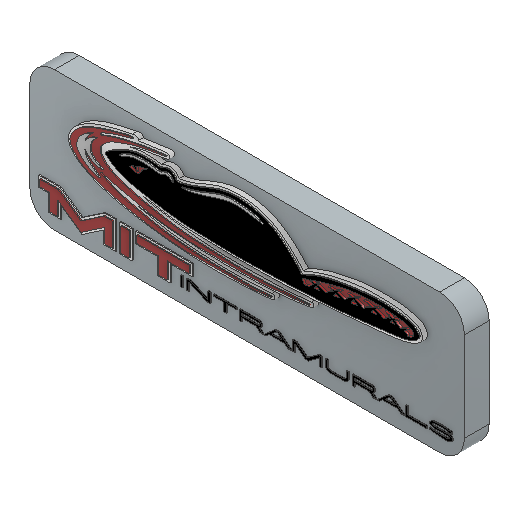
# Autodesk Inventor part: MIT Intramurals Banner
Saved by Autodesk Inventor 2026.2 (Build 302298000, 298)
## iProperties
Created: 2025-12-23
Part Number: MIT Intramurals Banner
Material: Generic
Document SubType Name: Modeling
Designer: andyeske
Density: 1 g/cm^3
Appearance: Default
Author: andyeske
Autodesk Inventor part; units mm, degrees
(part 1 of 2)
ref_plane "YZ Plane" through (0, 0, 0) normal (1, 0, 0) x (0, 1, 0)
ref_plane "XZ Plane" through (0, 0, 0) normal (0, 1, 0) x (-1, 0, 0)
ref_plane "XY Plane" through (0, 0, 0) normal (0, 0, 1) x (1, 0, 0)
sketch "Sketch1" plane through (0, 0, 0) normal (0, 0, 1) x (1, 0, 0)
  line L0 (-102.5583, 25.4534) -> (110.5342, 25.4534) construction
  line L1 (110.5342, 25.4534) -> (110.5342, -35.8107) construction
  line L2 (110.5342, -35.8107) -> (-102.5583, -35.8107) construction
  line L3 (-102.5583, -35.8107) -> (-102.5583, 25.4534) construction
  line L4 (-102.5583, 25.4534) -> (110.5342, 25.4534) construction
  line L5 (110.5342, 25.4534) -> (110.5342, -35.8107) construction
  line L6 (110.5342, -35.8107) -> (-102.5583, -35.8107) construction
  line L7 (-102.5583, -35.8107) -> (-102.5583, 25.4534) construction
  line L8 (-102.5583, -5.1786) -> (110.5342, -5.1786) construction
  line L9 (-107.6383, -40.8907) -> (115.6142, -40.8907)
  line L10 (115.6142, -40.8907) -> (115.6142, 30.5334)
  line L11 (115.6142, 30.5334) -> (-107.6383, 30.5334)
  line L12 (-107.6383, 30.5334) -> (-107.6383, -40.8907)
  line L13 (-107.6383, -40.8907) -> (115.6142, 30.5334) construction
  line L14 (115.6142, -40.8907) -> (-107.6383, 30.5334) construction
  spline S0 degree 4 poles (-52.4492, 24.3714) (-58.8702, 22.9595) (-67.573, 21.6476) (-80.0555, 16.5547) (-86.0471, 8.2755) (-85.3196, 1.057) (-71.5894, -7.0587) (-54.9195, -10.8267) (-25.8271, -15.277) (-1.6342, -15.5021) (17.3081, -13.4799) (19.6488, -13.3581) knots 0 0 0 0 0 0.204161 0.274872 0.345733 0.425063 0.520803 0.635182 0.756576 1 1 1 1 1
  spline S1 degree 4 poles (-49.0567, -6.4057) (-39.7782, -7.8854) (-36.8573, -10.6647) (4.3156, -12.1007) (6.0375, -11.212) (19.2729, -10.6088) knots 0 0 0 0 0 0.481309 1 1 1 1 1
  spline S2 degree 4 poles (-48.9231, -6.0144) (-47.2856, -6.3603) (-30.209, -9.1125) (-6.7858, -10.1005) (21.0365, -9.6313) (34.1993, -7.9209) (39.788, -6.6471) knots 0 0 0 0 0 0.386042 0.578559 1 1 1 1 1
  spline S3 degree 4 poles (-46.5779, -0.655) (-43.8171, -2.1998) (-20.6221, -4.7597) (-12.4054, -6.1125) (7.8539, -5.9766) (21.1432, -5.4197) (30.3375, -5.6283) (37.164, -4.3462) (39.6442, -4.2865) knots 0 0 0 0 0 0.358399 0.500414 0.629553 0.752083 1 1 1 1 1
  spline S4 degree 4 poles (-46.5779, -0.428) (-40.6413, -0.834) (-35.092, -3.6944) (-11.838, -3.5836) (9.8953, -4.1536) (37.76, -3.0641) (49.5551, -1.9589) (82.2104, 0.7181) (92.0004, 2.7859) (96.3774, 6.0719) (96.9345, 8.5326) (95.573, 12.2204) (91.8952, 13.5262) (86.96, 14.8593) (82.3457, 15.5732) (74.0371, 15.7321) (67.2255, 15.6466) (59.1842, 14.6025) (48.4661, 12.069) (45.437, 11.6483) (35.3646, 7.4843) (35.471, 7.4588) knots 0 0 0 0 0 0.13521 0.204072 0.278186 0.357458 0.429675 0.488839 0.535364 0.566154 0.593435 0.622619 0.655256 0.692209 0.732593 0.775833 0.821274 0.864817 0.909076 1 1 1 1 1
  spline S5 degree 4 poles (35.471, 7.4588) (32.9093, 10.589) (24.1083, 20.0316) (15.0532, 23.4669) (4.122, 25.3465) (-4.4474, 24.7856) (-11.5501, 22.5181) (-21.6412, 18.1562) (-21.1605, 18.2177) (-27.5995, 16.4904) (-28.3232, 16.6931) knots 0 0 0 0 0 0.300543 0.415952 0.52752 0.636808 0.734219 0.82255 1 1 1 1 1
  spline S6 degree 4 poles (-28.3232, 16.6931) (-29.0007, 17.4703) (-29.5286, 18.6185) (-32.267, 20.3015) (-35.437, 19.4052) (-36.852, 18.6173) (-37.322, 18.4594) knots 0 0 0 0 0 0.41933 0.600199 1 1 1 1 1
  spline S7 degree 4 poles (-37.322, 18.4594) (-38.5691, 18.5544) (-43.1872, 19.8396) (-49.0015, 18.9635) (-52.3655, 18.5024) (-53.4631, 18.0644) knots 0 0 0 0 0 0.521417 1 1 1 1 1
  spline S8 degree 4 poles (-53.5099, 18.2245) (-50.9519, 19.1283) (-47.5068, 20.3499) (-40.9121, 20.7668) (-34.7831, 22.3278) (-33.7292, 22.3321) (-33.0986, 23.0952) (-32.9733, 24.2409) (-33.4725, 24.8827) (-35.3883, 25.1437) (-39.835, 24.1062) (-46.9335, 23.5297) (-47.4631, 23.1662) (-49.3709, 23.0321) knots 0 0 0 0 0 0.266365 0.357545 0.430443 0.483452 0.524772 0.568835 0.624773 0.699993 0.786792 1 1 1 1 1
  spline S9 degree 4 poles (-49.3709, 23.0321) (-49.3469, 23.256) (-49.3072, 24.335) (-49.9777, 24.9683) (-51.9566, 24.5536) (-52.4492, 24.3714) knots 0 0 0 0 0 0.425634 1 1 1 1 1
  arc A0 (19.6488, -13.3581) -> (19.2729, -10.6088) centre (19.4518, -11.9847) ccw
  arc A1 (39.788, -6.6471) -> (39.6442, -4.2865) centre (39.6727, -5.4694) ccw
  arc A2 (-48.9231, -6.0144) -> (-49.0567, -6.4057) centre (-48.9661, -6.2182) ccw
  arc A3 (-46.5779, -0.428) -> (-46.5779, -0.655) centre (-46.5512, -0.5415) ccw
  arc A4 (-53.5099, 18.2245) -> (-53.4631, 18.0644) centre (-53.4821, 18.1458) ccw
  spline S10 degree 4 poles (-71.97, 15.4745) (-73.5618, 14.8176) (-78.0389, 12.5988) (-80.1652, 8.5391) (-80.3177, 3.0778) (-71.7488, -2.2177) (-71.8816, -1.1731) (-68.0997, -2.6081) knots 0 0 0 0 0 0.349269 0.493319 0.634154 1 1 1 1 1
  spline S11 degree 3 poles (-71.97, 15.4745) (-73.2885, 14.039) (-75.2326, 12.8836) (-75.6158, 10.3382) knots 0 0 0 0 1 1 1 1
  spline S12 degree 3 poles (-75.6158, 10.3382) (-74.6308, 12.2137) (-72.1942, 13.8735) (-69.6154, 14.6163) knots 0 0 0 0 1 1 1 1
  spline S13 degree 4 poles (-69.6154, 14.6163) (-70.4759, 13.8231) (-72.3788, 12.3221) (-73.059, 10.2756) (-73.1664, 5.2191) (-69.7067, 3.7408) (-68.2199, 2.6138) (-66.4762, 1.8118) knots 0 0 0 0 0 0.339065 0.480526 0.625412 1 1 1 1 1
  spline S14 degree 4 poles (-75.8015, 6.7353) (-74.6191, 4.6802) (-72.4475, 2.5037) (-68.6605, 1.822) (-66.4762, 1.8118) knots 0 0 0 0 0 1 1 1 1 1
  spline S15 degree 4 poles (-75.8015, 6.7353) (-75.5788, 4.044) (-75.7088, 2.5492) (-69.058, -1.4354) (-68.0997, -2.6081) knots 0 0 0 0 0 1 1 1 1 1
  spline S16 degree 4 poles (-52.048, 23.4288) (-54.2401, 23.3528) (-66.6857, 19.9381) (-79.4427, 16.3789) (-84.3823, 7.744) (-84.209, 4.7623) (-78.8244, -2.3227) (-66.6046, -6.5374) (-51.6417, -10.096) (-41.0552, -11.7905) (-18.7063, -14.7429) (-1.7175, -12.2275) (3.8289, -14.3334) (19.2729, -12.2118) knots 0 0 0 0 0 0.18081 0.244398 0.299004 0.356886 0.425964 0.50631 0.595714 0.686149 0.771857 1 1 1 1 1
  spline S17 degree 4 poles (-51.972, 22.8466) (-57.6402, 21.3754) (-58.1641, 21.4536) (-67.5415, 18.1413) (-68.4686, 17.0097) knots 0 0 0 0 0 1 1 1 1 1
  spline S18 degree 4 poles (-67.7151, 16.4274) (-64.426, 17.854) (-60.1317, 19.3505) (-45.9619, 22.8498) (-40.2437, 23.0375) (-34.715, 23.8652) knots 0 0 0 0 0 0.467692 1 1 1 1 1
  spline S19 degree 4 poles (-34.6772, 23.4704) (-38.4839, 22.7648) (-40.4639, 22.3554) (-50.7282, 21.246) (-60.3841, 16.8007) (-62.8171, 16.4662) (-68.298, 12.2075) (-69.5248, 8.3693) (-64.0493, 2.7683) (-55.3104, -0.0117) (-47.7069, -2.169) (-33.9304, -4.8768) (-23.6731, -6.2287) (-9.6141, -6.7589) (3.746, -7.4013) (15.6562, -7.092) (30.638, -6.3684) (37.5145, -5.6068) (39.0554, -5.469) knots 0 0 0 0 0 0.119852 0.168842 0.217962 0.26068 0.302266 0.349885 0.400894 0.460541 0.525181 0.593374 0.664659 0.734215 0.804927 0.871867 1 1 1 1 1
  spline S20 degree 4 poles (39.108, -5.7709) (37.4385, -6.308) (23.1011, -7.5786) (13.1163, -8.7313) (-7.0091, -8.2583) (-21.4952, -8.578) (-29.5439, -7.3415) (-41.2987, -6.7959) (-48.8299, -4.501) (-65.2605, -1.3176) (-67.5791, 0.1162) knots 0 0 0 0 0 0.240077 0.356564 0.466749 0.569739 0.662256 0.754281 1 1 1 1 1
  spline S21 degree 4 poles (-68.0997, -0.655) (-62.5259, -3.4157) (-61.765, -4.6975) (-42.4071, -9.0657) (-34.3124, -10.69) (-17.9846, -11.881) (-11.8888, -12.3355) (4.7444, -12.3507) (10.0463, -12.6177) (17.9731, -11.9242) (19.2729, -11.797) knots 0 0 0 0 0 0.246404 0.35873 0.472789 0.584911 0.695079 0.795942 1 1 1 1 1
  arc A5 (19.2729, -12.2118) -> (19.2729, -11.797) centre (19.2444, -12.0044) ccw
  arc A6 (-67.5791, 0.1162) -> (-68.0997, -0.655) centre (-67.7515, -0.3288) ccw
  arc A7 (39.108, -5.7709) -> (39.0554, -5.469) centre (39.0691, -5.6221) ccw
  arc A8 (-51.972, 22.8466) -> (-52.048, 23.4288) centre (-52.0378, 23.1341) ccw
  arc A9 (-34.6772, 23.4704) -> (-34.715, 23.8652) centre (-34.6856, 23.6688) ccw
  spline S22 degree 4 poles (-65.879, 9.2635) (-65.8749, 11.3275) (-55.3373, 15.7109) (-53.6712, 18.2111) (-38.9955, 17.9177) (-37.405, 16.714) (-33.7493, 19.5352) (-31.3534, 18.3976) (-29.5789, 16.7809) (-29.4647, 15.575) knots 0 0 0 0 0 0.357646 0.495506 0.61467 0.716133 0.79801 1 1 1 1 1
  spline S23 degree 4 poles (-29.4647, 15.575) (-28.1519, 15.0835) (-24.5872, 15.8727) (-18.5009, 18.1038) (-12.5083, 20.6718) (-6.1161, 23.2421) (3.0018, 24.3814) (11.5231, 23.0257) (21.4229, 19.5107) (27.5772, 14.3886) (34.927, 6.7369) (34.8654, 5.7735) knots 0 0 0 0 0 0.174571 0.259653 0.353316 0.452487 0.556196 0.662312 0.769869 1 1 1 1 1
  spline S24 degree 4 poles (34.8654, 5.7735) (40.8292, 8.1161) (40.6549, 10.0927) (71.7532, 15.7804) (83.2327, 13.7336) (92.5145, 13.0285) (96.6582, 8.6519) (94.223, 5.852) (89.2683, 3.6409) (84.9003, 2.9408) (72.4496, 1.6108) (62.4885, 0.1154) (50.6338, -0.6616) (26.6259, -2.1909) (16.6731, -2.1299) (2.2887, -2.9635) (-18.4876, -2.0158) (-30.9684, -1.9125) (-54.5772, 2.6604) (-59.4474, 3.6818) (-65.879, 9.2635) knots 0 0 0 0 0 0.126651 0.181647 0.230811 0.266967 0.298491 0.327835 0.362864 0.404742 0.452577 0.510294 0.568494 0.62822 0.690828 0.748447 0.808493 0.867431 1 1 1 1 1
  spline S25 degree 4 poles (-58.3596, 12.6825) (-57.2325, 13.7843) (-51.9107, 17.5748) (-41.5573, 16.8573) (-38.56, 15.7519) (-36.7348, 15.5391) (-35.2387, 16.9945) (-32.33, 17.386) (-31.3664, 15.6515) (-30.3695, 15.3825) (-30.6352, 13.9476) knots 0 0 0 0 0 0.357484 0.480034 0.576415 0.657357 0.736723 0.814996 1 1 1 1 1
  spline S26 degree 4 poles (-30.6352, 13.9476) (-30.9382, 14.2243) (-32.1883, 16.178) (-34.3185, 16.1348) (-36.0839, 15.0225) (-37.1207, 14.3376) (-39.694, 14.8986) (-41.6476, 15.3507) (-45.7698, 15.473) (-50.3637, 15.66) (-54.9604, 14.1617) (-57.2368, 12.3666) (-58.3596, 12.6825) knots 0 0 0 0 0 0.170055 0.237891 0.305971 0.377561 0.459955 0.555332 0.659577 0.768342 1 1 1 1 1
  spline S27 degree 4 poles (-26.2639, 14.356) (-23.3906, 14.8149) (-14.9027, 16.789) (-5.1775, 24.2035) (8.399, 20.9689) (12.1626, 21.0227) (15.3623, 18.6573) knots 0 0 0 0 0 0.432201 0.610065 1 1 1 1 1
  spline S28 degree 4 poles (15.3623, 18.6573) (14.0844, 19.1095) (6.0457, 20.2504) (1.0033, 21.6252) (-13.688, 16.6903) (-14.6354, 16.5131) (-24.8081, 13.4817) (-26.2639, 14.356) knots 0 0 0 0 0 0.34942 0.500031 0.649154 1 1 1 1 1
  spline S29 degree 2 poles (-53.3008, 9.911) (-52.5867, 10.6807) (-51.5889, 11.0921) knots 0 0 0 1 1 1
  line L15 (-51.5889, 11.0921) -> (-49.9017, 9.2326)
  line L16 (-49.9017, 9.2326) -> (-50.0556, 11.6422)
  spline S30 degree 3 poles (-50.0556, 11.6422) (-48.6963, 12.1055) (-46.1374, 12.8984) (-44.3311, 13.1726) knots 0 0 0 0 1 1 1 1
  spline S31 degree 3 poles (-44.3311, 13.1726) (-45.5318, 12.4854) (-46.2357, 11.5206) (-47.2677, 11.1827) knots 0 0 0 0 1 1 1 1
  spline S32 degree 4 poles (-47.2677, 11.1827) (-47.3636, 10.8042) (-47.2649, 10.0321) (-49.615, 8.1093) (-50.6841, 8.6477) (-52.7122, 9.4891) (-53.3008, 9.911) knots 0 0 0 0 0 0.361372 0.533494 1 1 1 1 1
  line L17 (35.2952, 4.3814) -> (36.3498, 1.9636)
  spline S33 degree 2 poles (35.2952, 4.3814) (37.0043, 5.036) (38.6042, 5.5033) knots 0 0 0 1 1 1
  spline S34 degree 2 poles (36.3498, 1.9636) (37.741, 2.2189) (38.9714, 2.5521) knots 0 0 0 1 1 1
  spline S35 degree 2 poles (38.9714, 2.5521) (39.7159, 3.5541) (41.2291, 4.6206) knots 0 0 0 1 1 1
  spline S36 degree 2 poles (38.6042, 5.5033) (40.0266, 5.3532) (41.2291, 4.6206) knots 0 0 0 1 1 1
  spline S37 degree 2 poles (39.2749, 5.685) (40.8676, 5.5413) (42.1574, 5.2848) knots 0 0 0 1 1 1
  spline S38 degree 4 poles (39.2749, 5.685) (40.1857, 6.0134) (43.263, 7.1325) (47.2971, 8.314) (55.8577, 10.4813) (59.3016, 11.343) (70.558, 12.3008) (76.0447, 12.4509) (85.7728, 11.2662) (89.5634, 10.9909) (92.783, 8.8272) (92.8791, 7.6694) (92.0215, 6.1081) (89.9165, 5.6648) (89.4278, 5.5033) knots 0 0 0 0 0 0.162413 0.243574 0.336675 0.435958 0.540053 0.643161 0.731074 0.799741 0.849228 0.891651 1 1 1 1 1
  spline S39 degree 3 poles (89.4278, 5.5033) (90.0048, 6.3278) (88.6176, 6.9599) (87.5827, 7.1374) knots 0 0 0 0 1 1 1 1
  spline S40 degree 2 poles (87.5827, 7.1374) (88.251, 8.0136) (89.9993, 8.7444) knots 0 0 0 1 1 1
  spline S41 degree 3 poles (89.9993, 8.7444) (89.0353, 9.1151) (87.0785, 8.2126) (85.9445, 7.2852) knots 0 0 0 0 1 1 1 1
  spline S42 degree 2 poles (85.9445, 7.2852) (85.1544, 8.1452) (82.7618, 9.2635) knots 0 0 0 1 1 1
  spline S43 degree 2 poles (82.7618, 9.2635) (83.5886, 10.0911) (85.0626, 10.3382) knots 0 0 0 1 1 1
  spline S44 degree 2 poles (85.0626, 10.3382) (83.7496, 10.5873) (81.9313, 9.718) knots 0 0 0 1 1 1
  spline S45 degree 3 poles (81.9313, 9.718) (80.9342, 10.2789) (79.3639, 10.9061) (77.8217, 11.0035) knots 0 0 0 0 1 1 1 1
  spline S46 degree 3 poles (77.8217, 11.0035) (78.7555, 10.5207) (80.1921, 9.8801) (80.6667, 9.2635) knots 0 0 0 0 1 1 1 1
  spline S47 degree 3 poles (80.6667, 9.2635) (78.9368, 8.8382) (78.6712, 8.3465) (77.423, 7.4588) knots 0 0 0 0 1 1 1 1
  spline S48 degree 2 poles (80.6667, 7.5944) (80.9598, 8.3322) (81.6868, 8.7444) knots 0 0 0 1 1 1
  spline S49 degree 2 poles (81.6868, 8.7444) (82.2926, 8.3928) (82.8551, 7.5944) knots 0 0 0 1 1 1
  line L18 (80.6667, 7.5944) -> (82.8551, 7.5944)
  line L19 (70.7025, 7.1374) -> (73.8247, 7.2162)
  line L20 (60.3527, 5.9944) -> (63.8972, 6.3408)
  line L21 (51.5538, 4.7315) -> (54.4025, 5.2848)
  line L22 (41.6408, 3.0069) -> (44.1266, 3.4055)
  spline S50 degree 2 poles (41.6408, 3.0069) (41.951, 3.9202) (42.3855, 4.2937) knots 0 0 0 1 1 1
  spline S51 degree 2 poles (42.3855, 4.2937) (43.4958, 4.1245) (44.1266, 3.4055) knots 0 0 0 1 1 1
  spline S52 degree 2 poles (42.1574, 5.2848) (43.1477, 6.2989) (44.8399, 7.0186) knots 0 0 0 1 1 1
  spline S53 degree 2 poles (44.8399, 7.0186) (43.7611, 6.1187) (43.1407, 5.2848) knots 0 0 0 1 1 1
  spline S54 degree 3 poles (43.1407, 5.2848) (44.4101, 5.0932) (46.3814, 4.5665) (47.5565, 4.0873) knots 0 0 0 0 1 1 1 1
  spline S55 degree 3 poles (47.5565, 4.0873) (48.3925, 4.8563) (50.3732, 6.2541) (51.2037, 6.5341) knots 0 0 0 0 1 1 1 1
  spline S56 degree 3 poles (51.2037, 6.5341) (50.1722, 6.995) (49.7103, 7.113) (48.5739, 7.2608) knots 0 0 0 0 1 1 1 1
  spline S57 degree 3 poles (48.5739, 7.2608) (49.332, 7.5631) (51.2725, 7.4257) (52.024, 7.099) knots 0 0 0 0 1 1 1 1
  spline S58 degree 3 poles (52.024, 7.099) (53.0571, 7.7103) (54.2865, 8.498) (55.7131, 8.7927) knots 0 0 0 0 1 1 1 1
  spline S59 degree 3 poles (55.7131, 8.7927) (54.9237, 8.3987) (53.6734, 7.6255) (53.2188, 7.0186) knots 0 0 0 0 1 1 1 1
  spline S60 degree 3 poles (53.2188, 7.0186) (53.9015, 6.9339) (55.7193, 6.6122) (56.9696, 5.685) knots 0 0 0 0 1 1 1 1
  spline S61 degree 2 poles (51.5538, 4.7315) (51.7348, 5.3219) (52.4733, 6.2312) knots 0 0 0 1 1 1
  spline S62 degree 2 poles (52.4733, 6.2312) (53.4059, 5.9476) (54.4025, 5.2848) knots 0 0 0 1 1 1
  spline S63 degree 2 poles (70.7025, 7.1374) (71.1539, 7.9459) (72.0142, 8.5077) knots 0 0 0 1 1 1
  spline S64 degree 2 poles (72.0142, 8.5077) (73.1907, 8.178) (73.8247, 7.2162) knots 0 0 0 1 1 1
  spline S65 degree 2 poles (60.3527, 5.9944) (60.8212, 7.1738) (61.7016, 8.0103) knots 0 0 0 1 1 1
  spline S66 degree 2 poles (61.7016, 8.0103) (63.1746, 7.5515) (63.8972, 6.3408) knots 0 0 0 1 1 1
  spline S67 degree 2 poles (56.9696, 5.685) (58.6077, 7.5518) (60.7559, 8.5077) knots 0 0 0 1 1 1
  spline S68 degree 2 poles (60.7559, 8.5077) (59.8431, 8.9671) (58.568, 9.2635) knots 0 0 0 1 1 1
  spline S69 degree 2 poles (58.568, 9.2635) (59.9688, 9.4306) (61.5188, 8.9027) knots 0 0 0 1 1 1
  spline S70 degree 2 poles (61.5188, 8.9027) (62.6832, 9.7229) (64.527, 10.2202) knots 0 0 0 1 1 1
  spline S71 degree 2 poles (64.527, 10.2202) (63.4518, 9.6666) (62.5551, 8.7927) knots 0 0 0 1 1 1
  spline S72 degree 3 poles (62.5551, 8.7927) (64.4258, 8.2771) (65.688, 7.6378) (66.7581, 6.7295) knots 0 0 0 0 1 1 1 1
  spline S73 degree 3 poles (66.7581, 6.7295) (67.8827, 7.847) (69.6665, 8.8024) (70.7025, 8.9027) knots 0 0 0 0 1 1 1 1
  spline S74 degree 3 poles (70.7025, 8.9027) (70.1912, 9.604) (68.038, 10.1459) (66.9267, 10.338) knots 0 0 0 0 1 1 1 1
  spline S75 degree 3 poles (66.9267, 10.338) (68.3767, 10.6734) (70.5215, 9.7878) (71.7293, 9.5928) knots 0 0 0 0 1 1 1 1
  spline S76 degree 3 poles (71.7293, 9.5928) (72.6223, 9.9336) (74.2672, 10.8902) (75.4899, 10.9318) knots 0 0 0 0 1 1 1 1
  spline S77 degree 3 poles (75.4899, 10.9318) (74.5963, 10.619) (73.0858, 9.6113) (72.8404, 9.2635) knots 0 0 0 0 1 1 1 1
  spline S78 degree 3 poles (72.8404, 9.2635) (74.6153, 8.8325) (75.731, 8.1456) (77.423, 7.4588) knots 0 0 0 0 1 1 1 1
  line L23 (-101.4437, -24.341) -> (-96.395, -24.341)
  line L24 (-96.395, -24.341) -> (-96.395, -32.9519)
  line L25 (-96.395, -32.9519) -> (-92.1637, -32.9519)
  line L26 (-92.1637, -32.9519) -> (-92.1637, -25.7224)
  line L27 (-92.1637, -25.7224) -> (-80.2835, -34.0057)
  line L28 (-80.2835, -34.0057) -> (-68.147, -25.7224)
  line L29 (-68.147, -25.7224) -> (-68.147, -33.1318)
  line L30 (-68.147, -33.1318) -> (-63.961, -33.1318)
  line L31 (-63.961, -33.1318) -> (-63.961, -20.8988)
  line L32 (-63.961, -20.8988) -> (-68.4676, -20.8988)
  line L33 (-68.4676, -20.8988) -> (-80.2835, -28.9632)
  line L34 (-80.2835, -28.9632) -> (-91.8499, -20.8988)
  line L35 (-91.8499, -20.8988) -> (-101.4437, -20.8988)
  line L36 (-101.4437, -20.8988) -> (-101.4437, -24.341)
  line L37 (-59.868, -20.8988) -> (-55.6283, -20.8988)
  line L38 (-55.6283, -20.8988) -> (-55.6283, -33.1318)
  line L39 (-55.6283, -33.1318) -> (-59.868, -33.1318)
  line L40 (-59.868, -33.1318) -> (-59.868, -20.8988)
  line L41 (-29.8009, -28.0712) -> (-28.5736, -28.0712)
  line L42 (-28.5736, -28.0712) -> (-28.5736, -33.1318)
  line L43 (-28.5736, -33.1318) -> (-29.8009, -33.1318)
  line L44 (-29.8009, -33.1318) -> (-29.8009, -28.0712)
  line L45 (-51.7454, -20.8988) -> (-51.7454, -24.6191)
  line L46 (-51.7454, -24.6191) -> (-40.4236, -24.6191)
  line L47 (-40.4236, -24.6191) -> (-40.4236, -33.1318)
  line L48 (-40.4236, -33.1318) -> (-36.0253, -33.1318)
  line L49 (-36.0253, -33.1318) -> (-36.0253, -24.6191)
  line L50 (-36.0253, -24.6191) -> (-24.5946, -24.6191)
  line L51 (-24.5946, -24.6191) -> (-24.5946, -20.8988)
  line L52 (-24.5946, -20.8988) -> (-51.7454, -20.8988)
  line L53 (-26.5667, -28.0712) -> (-26.5667, -33.1318)
  line L54 (-26.5667, -33.1318) -> (-25.4696, -33.1318)
  line L55 (-25.4696, -33.1318) -> (-25.4696, -28.9632)
  line L56 (-25.4696, -28.9632) -> (-16.0059, -33.1318)
  line L57 (-16.0059, -33.1318) -> (-14.4445, -33.1318)
  line L58 (-14.4445, -33.1318) -> (-14.4445, -28.0712)
  line L59 (-14.4445, -28.0712) -> (-15.7205, -28.0712)
  line L60 (-15.7205, -28.0712) -> (-15.7205, -31.9239)
  line L61 (-15.7205, -31.9239) -> (-24.4669, -28.0712)
  line L62 (-24.4669, -28.0712) -> (-26.5667, -28.0712)
  line L63 (-12.884, -28.0712) -> (-0.8389, -28.0712)
  line L64 (-0.8389, -28.0712) -> (-0.8389, -28.9632)
  line L65 (-0.8389, -28.9632) -> (-6.1614, -28.9632)
  line L66 (-6.1614, -28.9632) -> (-6.1614, -33.1318)
  line L67 (-6.1614, -33.1318) -> (-7.5308, -33.1318)
  line L68 (-7.5308, -33.1318) -> (-7.5308, -28.9632)
  line L69 (-7.5308, -28.9632) -> (-12.884, -28.9632)
  line L70 (-12.884, -28.9632) -> (-12.884, -28.0712)
  line L71 (0.5155, -28.0712) -> (0.5155, -33.1318)
  line L72 (0.5155, -33.1318) -> (1.6717, -33.1318)
  line L73 (1.6717, -33.1318) -> (1.6717, -31.3271)
  line L74 (1.6717, -31.3271) -> (9.09, -31.3271)
  line L75 (9.09, -31.3271) -> (11.1121, -33.1318)
  line L76 (11.1121, -33.1318) -> (12.6994, -33.1318)
  line L77 (12.6994, -33.1318) -> (10.6774, -31.3271)
  line L78 (0.5155, -28.0712) -> (10.6774, -28.0712)
  line L79 (10.4286, -29.1342) -> (1.6717, -29.1342)
  line L80 (1.6717, -29.1342) -> (1.6717, -30.3018)
  line L81 (1.6717, -30.3018) -> (10.4286, -30.3018)
  arc A10 (10.4286, -30.3018) -> (10.4286, -29.1342) centre (10.3913, -29.718) ccw
  arc A11 (10.6774, -31.3271) -> (10.6774, -28.0712) centre (10.2386, -29.6991) ccw
  line L82 (12.9309, -33.1318) -> (18.7874, -28.0712)
  line L83 (18.7874, -28.0712) -> (20.8265, -28.0712)
  line L84 (20.8265, -28.0712) -> (27.1651, -33.1318)
  line L85 (27.1651, -33.1318) -> (25.5653, -33.1318)
  line L86 (25.5653, -33.1318) -> (23.734, -31.6698)
  line L87 (23.734, -31.6698) -> (15.8591, -31.6698)
  line L88 (15.8591, -31.6698) -> (14.1671, -33.1318)
  line L89 (14.1671, -33.1318) -> (12.9309, -33.1318)
  line L90 (17.1877, -30.7607) -> (22.4353, -30.7607)
  line L91 (22.4353, -30.7607) -> (20.4209, -28.798)
  line L92 (20.4209, -28.798) -> (19.4154, -28.798)
  line L93 (19.4154, -28.798) -> (17.1877, -30.7607)
  line L94 (172.9021, -50.0972) -> (-40.1904, -50.0972) construction
  line L95 (172.9021, -50.0972) -> (-40.1904, -50.0972) construction
  line L96 (58.6314, -28.0318) -> (58.6314, -33.0923)
  line L97 (58.6314, -33.0923) -> (59.7876, -33.0923)
  line L98 (59.7876, -33.0923) -> (59.7876, -31.2876)
  line L99 (59.7876, -31.2876) -> (67.2059, -31.2876)
  line L100 (67.2059, -31.2876) -> (69.228, -33.0923)
  line L101 (69.228, -33.0923) -> (70.8153, -33.0923)
  line L102 (70.8153, -33.0923) -> (68.7933, -31.2876)
  line L103 (58.6314, -28.0318) -> (68.7933, -28.0318)
  line L104 (68.5445, -29.0947) -> (59.7876, -29.0947)
  line L105 (59.7876, -29.0947) -> (59.7876, -30.2624)
  line L106 (59.7876, -30.2624) -> (68.5445, -30.2624)
  arc A12 (68.5445, -30.2624) -> (68.5445, -29.0947) centre (68.5073, -29.6785) ccw
  arc A13 (68.7933, -31.2876) -> (68.7933, -28.0318) centre (68.3545, -29.6597) ccw
  line L107 (71.0468, -33.0923) -> (76.9033, -28.0318)
  line L108 (76.9033, -28.0318) -> (78.9424, -28.0318)
  line L109 (78.9424, -28.0318) -> (85.281, -33.0923)
  line L110 (85.281, -33.0923) -> (83.6812, -33.0923)
  line L111 (83.6812, -33.0923) -> (81.8499, -31.6303)
  line L112 (81.8499, -31.6303) -> (73.975, -31.6303)
  line L113 (73.975, -31.6303) -> (72.2831, -33.0923)
  line L114 (72.2831, -33.0923) -> (71.0468, -33.0923)
  line L115 (75.3036, -30.7212) -> (80.5512, -30.7212)
  line L116 (80.5512, -30.7212) -> (78.5369, -28.7586)
  line L117 (78.5369, -28.7586) -> (77.5313, -28.7586)
  line L118 (77.5313, -28.7586) -> (75.3036, -30.7212)
  line L119 (27.6953, -33.0923) -> (27.6953, -28.0318)
  line L120 (27.6953, -28.0318) -> (29.6369, -28.0318)
  line L121 (29.6369, -28.0318) -> (35.2952, -32.19)
  line L122 (35.2952, -32.19) -> (41.2291, -28.0318)
  line L123 (41.2291, -28.0318) -> (42.8837, -28.0318)
  line L124 (42.8837, -28.0318) -> (42.8837, -33.0923)
  line L125 (42.8837, -33.0923) -> (41.6408, -33.0923)
  line L126 (41.6408, -33.0923) -> (41.6408, -29.0947)
  line L127 (41.6408, -29.0947) -> (36.1117, -33.3551)
  line L128 (36.1117, -33.3551) -> (34.439, -33.3551)
  line L129 (34.439, -33.3551) -> (29.0483, -29.1342)
  line L130 (29.0483, -29.1342) -> (29.0483, -33.0923)
  line L131 (29.0483, -33.0923) -> (27.6953, -33.0923)
  line L132 (44.5357, -28.0318) -> (45.8846, -28.0318)
  line L133 (44.5357, -28.0318) -> (44.5357, -31.2446)
  line L134 (45.8846, -28.0318) -> (45.8846, -31.2446)
  line L135 (55.4313, -31.1132) -> (55.4313, -28.0318)
  line L136 (55.4313, -28.0318) -> (56.7534, -28.0318)
  line L137 (56.7534, -28.0318) -> (56.7534, -31.1132)
  line L138 (47.9942, -32.19) -> (53.8931, -32.19)
  line L139 (47.4288, -33.0923) -> (54.2843, -33.0923)
  spline S79 degree 2 poles (45.8846, -31.2446) (46.106, -31.8542) (47.9942, -32.19) knots 0 0 0 1 1 1
  spline S80 degree 3 poles (44.5357, -31.2446) (44.5599, -32.2303) (45.931, -32.9686) (47.4288, -33.0923) knots 0 0 0 0 1 1 1 1
  spline S81 degree 3 poles (56.7534, -31.1132) (56.7847, -31.9085) (55.4171, -32.9141) (54.2843, -33.0923) knots 0 0 0 0 1 1 1 1
  spline S82 degree 2 poles (53.8931, -32.19) (55.2787, -31.9913) (55.4313, -31.1132) knots 0 0 0 1 1 1
  line L140 (85.9445, -28.0712) -> (87.1046, -28.0712)
  line L141 (87.1046, -28.0712) -> (87.1046, -31.9938)
  line L142 (87.1046, -31.9938) -> (96.8774, -31.9938)
  line L143 (96.8774, -31.9938) -> (96.8774, -33.0869)
  line L144 (96.8774, -33.0869) -> (85.9445, -33.0869)
  line L145 (85.9445, -33.0869) -> (85.9445, -28.0712)
  line L146 (98.2674, -31.6303) -> (98.2674, -32.5404)
  line L147 (109.6722, -28.4037) -> (109.6722, -29.3372)
  spline S83 degree 4 poles (109.6722, -28.4037) (108.7733, -28.0929) (105.6478, -27.7752) (103.1637, -27.669) (99.2636, -27.9958) (98.2311, -28.988) (98.1711, -29.9388) (99.4289, -31.0631) (101.7371, -30.9908) (105.1225, -30.9191) (107.0954, -30.7922) (108.598, -31.0126) (108.829, -31.6343) (107.9042, -32.2349) (105.4491, -32.1575) (101.0474, -32.2825) (98.7105, -31.9386) (98.2674, -31.6303) knots 0 0 0 0 0 0.176908 0.243948 0.300203 0.348723 0.396841 0.456186 0.523231 0.589094 0.644157 0.685091 0.722698 0.771731 0.835847 1 1 1 1 1
  spline S84 degree 4 poles (98.2674, -32.5404) (99.5553, -33.0936) (102.1491, -32.7939) (106.7339, -33.9297) (110.1842, -32.5353) (110.0663, -30.5611) (108.6148, -30.0593) (106.1535, -29.9773) (102.3534, -29.9259) (101.0004, -30.198) (99.2528, -29.843) (99.5332, -29.1911) (100.6421, -28.7892) (102.2414, -28.7031) (108.031, -28.4051) (107.7183, -29.2242) (109.6722, -29.3372) knots 0 0 0 0 0 0.193476 0.265024 0.326054 0.382919 0.447483 0.515446 0.581924 0.636535 0.67795 0.716326 0.766204 0.827883 1 1 1 1 1
  point P0 (0, 0)
  point P1 (3.9879, -5.1786)
  point P2 (-63.2696, 21.994)
  point P3 (-74.1898, 18.163)
  point P4 (-81.9273, 13.059)
  point P5 (-84.9907, 8.2462)
  point P6 (-84.46, 3.2243)
  point P7 (-75.3767, -4.2012)
  point P8 (-57.1798, -10.0522)
  point P9 (-32.848, -13.7119)
  point P10 (-6.16, -14.8406)
  point P11 (14.2841, -13.7934)
  point P12 (-39.1333, -8.3929)
  point P13 (-27.998, -10.0579)
  point P14 (-7.53, -11.2991)
  point P15 (5.0636, -11.3252)
  point P16 (-44.3448, -6.768)
  point P17 (-26.9622, -8.7993)
  point P18 (-6.5969, -9.7072)
  point P19 (14.2529, -9.4349)
  point P20 (30.7774, -8.1445)
  point P21 (-35.1237, -2.9829)
  point P22 (-16.8054, -5.1786)
  point P23 (-5.2292, -5.9063)
  point P24 (8.4022, -5.8766)
  point P25 (19.2472, -5.6046)
  point P26 (28.0274, -5.3492)
  point P27 (35.4082, -4.6884)
  point P28 (-39.5981, -1.5241)
  point P29 (-29.3179, -3.0262)
  point P30 (-10.4174, -3.7442)
  point P31 (10.1672, -3.8571)
  point P32 (34.8638, -3.027)
  point P33 (55.2915, -1.5051)
  point P34 (86.7801, 1.9619)
  point P35 (94.0802, 4.6158)
  point P36 (96.2193, 6.7261)
  point P37 (96.5848, 8.6266)
  point P38 (95.4548, 11.3806)
  point P39 (92.3217, 13.2998)
  point P40 (87.6339, 14.5956)
  point P41 (82.6419, 15.3745)
  point P42 (74.8311, 15.6746)
  point P43 (67.1736, 15.4606)
  point P44 (58.757, 14.3443)
  point P45 (51.1193, 12.7384)
  point P46 (45.883, 11.3954)
  point P47 (37.7337, 8.4225)
  point P48 (28.8398, 14.3559)
  point P49 (19.2717, 21.1238)
  point P50 (11.5307, 23.8652)
  point P51 (3.988, 24.9481)
  point P52 (-4.4388, 24.3714)
  point P53 (-13.1968, 21.7075)
  point P54 (-19.5689, 19.0248)
  point P55 (-21.7475, 18.1683)
  point P56 (-25.4696, 17.1317)
  point P57 (-29.2255, 17.8447)
  point P58 (-30.4143, 18.919)
  point P59 (-32.3677, 19.6364)
  point P60 (-34.677, 19.4695)
  point P61 (-36.5087, 18.8078)
  point P62 (-39.5897, 18.8083)
  point P63 (-44.0219, 19.2144)
  point P64 (-48.7169, 18.9607)
  point P65 (-51.8224, 18.5106)
  point P66 (-49.593, 19.473)
  point P67 (-44.0257, 20.5822)
  point P68 (-37.3281, 21.7165)
  point P69 (-34.2972, 22.3327)
  point P70 (-33.6058, 22.6038)
  point P71 (-33.1785, 23.201)
  point P72 (-33.0815, 24.0917)
  point P73 (-33.3977, 24.6171)
  point P74 (-34.5396, 24.9508)
  point P75 (-37.937, 24.6046)
  point P76 (-44.4064, 23.7068)
  point P77 (-47.4349, 23.2658)
  point P78 (-49.3615, 23.457)
  point P79 (-49.507, 24.0557)
  point P80 (-49.9521, 24.4922)
  point P81 (-51.1056, 24.6434)
  point P82 (-75.3651, 13.6542)
  point P83 (-78.6663, 10.4705)
  point P84 (-79.9317, 7.4588)
  point P85 (-79.5771, 4.6205)
  point P86 (-75.3649, 0.4414)
  point P87 (-71.9699, -1.3673)
  point P88 (-73.3328, 14.1502)
  point P89 (-74.7076, 12.6095)
  point P90 (-74.3626, 11.9588)
  point P91 (-72.2711, 13.4977)
  point P92 (-71.1635, 13.1726)
  point P93 (-72.4276, 11.4007)
  point P94 (-72.9824, 9.2635)
  point P95 (-72.7429, 6.6215)
  point P96 (-71.1254, 4.6206)
  point P97 (-68.9349, 3.1442)
  point P98 (-74.3628, 4.8608)
  point P99 (-71.9701, 3.1442)
  point P100 (-68.9349, 2.0854)
  point P101 (-75.5006, 4.7315)
  point P102 (-74.197, 2.5521)
  point P103 (-70.5188, -0.655)
  point P104 (-58.7239, 21.9977)
  point P105 (-73.5666, 17.1317)
  point P106 (-81.6263, 11.7004)
  point P107 (-83.8633, 7.7029)
  point P108 (-83.7541, 5.2058)
  point P109 (-80.2835, 0.4416)
  point P110 (-68.2715, -5.7102)
  point P111 (-52.4492, -9.7219)
  point P112 (-40.4236, -11.7967)
  point P113 (-24.7819, -13.3581)
  point P114 (-9.9687, -13.3581)
  point P115 (0.5155, -13.3581)
  point P116 (-56.7595, 21.6078)
  point P117 (-61.1409, 20.2417)
  point P118 (-66.4828, 18.1506)
  point P119 (-63.5422, 18.0643)
  point P120 (-58.2102, 19.6365)
  point P121 (-49.7373, 21.6078)
  point P122 (-42.2214, 22.8773)
  point P123 (-39.0088, 22.688)
  point P124 (-44.1604, 21.8246)
  point P125 (-53.849, 19.4702)
  point P126 (-60.4408, 17.0103)
  point P127 (-63.4115, 15.692)
  point P128 (-67.4906, 12.238)
  point P129 (-68.4656, 8.903)
  point P130 (-64.8238, 4.2941)
  point P131 (-56.5431, 0.442)
  point P132 (-47.8855, -1.9428)
  point P133 (-35.1146, -4.5144)
  point P134 (-23.4273, -6.0139)
  point P135 (-9.4628, -6.7901)
  point P136 (3.6455, -7.2272)
  point P137 (14.2708, -7.0717)
  point P138 (27.697, -6.4046)
  point P139 (36.5356, -5.7101)
  point P140 (34.1531, -6.5046)
  point P141 (21.1076, -7.7405)
  point P142 (8.4273, -8.3923)
  point P143 (-8.2602, -8.3913)
  point P144 (-22.5807, -8.1408)
  point P145 (-30.4198, -7.4265)
  point P146 (-37.3263, -6.7895)
  point P147 (-44.6879, -5.5691)
  point P148 (-58.2119, -2.6075)
  point P149 (-62.2204, -3.5962)
  point P150 (-54.9765, -6.0145)
  point P151 (-41.9684, -9.083)
  point P152 (-32.8492, -10.6082)
  point P153 (-19.1084, -11.7956)
  point P154 (-10.3187, -12.2468)
  point P155 (1.436, -12.3955)
  point P156 (9.341, -12.3982)
  point P157 (16.2097, -12.0534)
  point P158 (-62.3675, 12.4616)
  point P159 (-54.6455, 16.2882)
  point P160 (-47.3018, 17.8448)
  point P161 (-38.691, 17.4215)
  point P162 (-36.7676, 17.498)
  point P163 (-34.4878, 18.5117)
  point P164 (-32.3678, 18.5117)
  point P165 (-30.4181, 17.2972)
  point P166 (-27.3478, 15.4745)
  point P167 (-23.0284, 16.5574)
  point P168 (-17.6943, 18.5119)
  point P169 (-12.884, 20.4848)
  point P170 (-6.5796, 22.6878)
  point P171 (2.6728, 23.8652)
  point P172 (11.5307, 22.6878)
  point P173 (18.7874, 20.0395)
  point P174 (25.5653, 15.575)
  point P175 (33.007, 8.4244)
  point P176 (40.3926, 8.2429)
  point P177 (51.1245, 11.4007)
  point P178 (75.4899, 14.356)
  point P179 (86.3018, 13.4979)
  point P180 (93.6234, 11.1826)
  point P181 (95.4681, 8.4244)
  point P182 (94.2289, 6.3408)
  point P183 (90.4018, 4.2937)
  point P184 (85.6918, 3.1442)
  point P185 (74.8418, 1.8118)
  point P186 (63.7317, 0.4416)
  point P187 (50.5345, -0.655)
  point P188 (27.6953, -1.9432)
  point P189 (15.9178, -2.2996)
  point P190 (1.9042, -2.6081)
  point P191 (-17.3795, -2.1379)
  point P192 (-29.4647, -1.3672)
  point P193 (-45.8141, 1.1119)
  point P194 (-57.401, 3.9682)
  point P195 (-55.083, 14.786)
  point P196 (-45.73, 16.766)
  point P197 (-39.8397, 16.1558)
  point P198 (-38.1212, 15.7642)
  point P199 (-36.7882, 15.8656)
  dimension "d6" = 5.08
  dimension "d10" = 5.08
  constraints: 286 end point, 46 perpendicular, 30 parallel, 28 point on circle, 28 point on line, 19 horizontal, 14 centre point, 8 vertical, 5 midpoint, 527 other
  measures "d6" distance between parallel lines of L0 L11
  measures "d10" distance between parallel lines of L1 L10
sketch "Sketch2" plane through (0, 0, 0) normal (0, 0, 1) x (1, 0, 0)
  line L0 (115.6142, 30.5334) -> (-107.6383, 30.5334) projected
  line L1 (-107.6383, 30.5334) -> (-107.6383, -40.8907) projected
  line L2 (-107.6383, -40.8907) -> (115.6142, -40.8907) projected
  line L3 (115.6142, -40.8907) -> (115.6142, 30.5334) projected
  point P0 (0, 0)
extrude "Extrusion1" add sketch "Sketch1" along normal blind 12.7 contours L12 L11 L10 L9 | S9 S8 A4 S7 S6 S5 S4 A3 S3 A1 S2 A2 S1 A0 S0 | S11 S12 S13 S14 S15 S10 | S22 S23 S24 | S25 S26 | S27 S28 | S29 L15 L16 S30 S31 S32 | S33 S36 S35 S34 L17 | S38 S39 S40 S41 S42 S43 S44 S45 S46 S47 S78 S77 S76 S75 S74 S73 S72 S71 S70 S69 S68 S67 S60 S59 S58 S57 S56 S55 S54 S53 S52 S37 | S48 S49 L18 | S63 S64 L19 | S65 S66 L20 | S61 S62 L21 | S50 S51 L22 | L36 L35 L34 L33 L32 L31 L30 L29 L28 L27 L26 L25 L24 L23 | L37 L38 L39 L40 | L41 L42 L43 L44 | L52 L51 L50 L49 L48 L47 L46 L45 | L62 L61 L60 L59 L58 L57 L56 L55 L54 L53 | L63 L64 L65 L66 L67 L68 L69 L70 | L78 A11 L77 L76 L75 L74 L73 L72 L71 | A10 L81 L80 L79 | L82 L83 L84 L85 L86 L87 L88 L89 | L93 L92 L91 L90 | L103 A13 L102 L101 L100 L99 L98 L97 L96 | A12 L106 L105 L104 | L107 L108 L109 L110 L111 L112 L113 L114 | L118 L117 L116 L115 | L119 L120 L121 L122 L123 L124 L125 L126 L127 L128 L129 L130 L131 | L132 L134 S79 L138 S82 L135 L136 L137 S81 L139 S80 L133 | L140 L141 L142 L143 L144 L145 | S83 L147 S84 L146
sketch "Sketch3" plane through (0, 0, 12.7) normal (0, 0, 1) x (1, 0, 0)
  spline S0 degree 4 poles (35.471, 7.4588) (32.9093, 10.589) (24.1083, 20.0316) (15.0532, 23.4669) (4.122, 25.3465) (-4.4474, 24.7856) (-11.5501, 22.5181) (-21.6412, 18.1562) (-21.1605, 18.2177) (-27.5995, 16.4904) (-28.3232, 16.6931) knots 0 0 0 0 0 0.300543 0.415952 0.52752 0.636808 0.734219 0.82255 1 1 1 1 1 projected
  spline S1 degree 4 poles (-46.5779, -0.428) (-40.6413, -0.834) (-35.092, -3.6944) (-11.838, -3.5836) (9.8953, -4.1536) (37.76, -3.0641) (49.5551, -1.9589) (82.2104, 0.7181) (92.0004, 2.7859) (96.3774, 6.0719) (96.9345, 8.5326) (95.573, 12.2204) (91.8952, 13.5262) (86.96, 14.8593) (82.3457, 15.5732) (74.0371, 15.7321) (67.2255, 15.6466) (59.1842, 14.6025) (48.4661, 12.069) (45.437, 11.6483) (35.3646, 7.4843) (35.471, 7.4588) knots 0 0 0 0 0 0.13521 0.204072 0.278186 0.357458 0.429675 0.488839 0.535364 0.566154 0.593435 0.622619 0.655256 0.692209 0.732593 0.775833 0.821274 0.864817 0.909076 1 1 1 1 1 projected
  arc A0 (-46.5779, -0.428) -> (-46.5779, -0.655) centre (-46.5512, -0.5415) ccw projected
  spline S2 degree 4 poles (-46.5779, -0.655) (-43.8171, -2.1998) (-20.6221, -4.7597) (-12.4054, -6.1125) (7.8539, -5.9766) (21.1432, -5.4197) (30.3375, -5.6283) (37.164, -4.3462) (39.6442, -4.2865) knots 0 0 0 0 0 0.358399 0.500414 0.629553 0.752083 1 1 1 1 1 projected
  arc A1 (39.788, -6.6471) -> (39.6442, -4.2865) centre (39.6727, -5.4694) ccw projected
  spline S3 degree 4 poles (-48.9231, -6.0144) (-47.2856, -6.3603) (-30.209, -9.1125) (-6.7858, -10.1005) (21.0365, -9.6313) (34.1993, -7.9209) (39.788, -6.6471) knots 0 0 0 0 0 0.386042 0.578559 1 1 1 1 1 projected
  arc A2 (-48.9231, -6.0144) -> (-49.0567, -6.4057) centre (-48.9661, -6.2182) ccw projected
  spline S4 degree 4 poles (-49.0567, -6.4057) (-39.7782, -7.8854) (-36.8573, -10.6647) (4.3156, -12.1007) (6.0375, -11.212) (19.2729, -10.6088) knots 0 0 0 0 0 0.481309 1 1 1 1 1 projected
  arc A3 (19.6488, -13.3581) -> (19.2729, -10.6088) centre (19.4518, -11.9847) ccw projected
  spline S5 degree 4 poles (-52.4492, 24.3714) (-58.8702, 22.9595) (-67.573, 21.6476) (-80.0555, 16.5547) (-86.0471, 8.2755) (-85.3196, 1.057) (-71.5894, -7.0587) (-54.9195, -10.8267) (-25.8271, -15.277) (-1.6342, -15.5021) (17.3081, -13.4799) (19.6488, -13.3581) knots 0 0 0 0 0 0.204161 0.274872 0.345733 0.425063 0.520803 0.635182 0.756576 1 1 1 1 1 projected
  spline S6 degree 4 poles (-49.3709, 23.0321) (-49.3469, 23.256) (-49.3072, 24.335) (-49.9777, 24.9683) (-51.9566, 24.5536) (-52.4492, 24.3714) knots 0 0 0 0 0 0.425634 1 1 1 1 1 projected
  spline S7 degree 4 poles (-53.5099, 18.2245) (-50.9519, 19.1283) (-47.5068, 20.3499) (-40.9121, 20.7668) (-34.7831, 22.3278) (-33.7292, 22.3321) (-33.0986, 23.0952) (-32.9733, 24.2409) (-33.4725, 24.8827) (-35.3883, 25.1437) (-39.835, 24.1062) (-46.9335, 23.5297) (-47.4631, 23.1662) (-49.3709, 23.0321) knots 0 0 0 0 0 0.266365 0.357545 0.430443 0.483452 0.524772 0.568835 0.624773 0.699993 0.786792 1 1 1 1 1 projected
  spline S8 degree 4 poles (-28.3232, 16.6931) (-29.0007, 17.4703) (-29.5286, 18.6185) (-32.267, 20.3015) (-35.437, 19.4052) (-36.852, 18.6173) (-37.322, 18.4594) knots 0 0 0 0 0 0.41933 0.600199 1 1 1 1 1 projected
  spline S9 degree 4 poles (-37.322, 18.4594) (-38.5691, 18.5544) (-43.1872, 19.8396) (-49.0015, 18.9635) (-52.3655, 18.5024) (-53.4631, 18.0644) knots 0 0 0 0 0 0.521417 1 1 1 1 1 projected
  arc A4 (-53.5099, 18.2245) -> (-53.4631, 18.0644) centre (-53.4821, 18.1458) ccw projected
  point P0 (0, 0)
  point P1 (35.47, 7.4601)
extrude "Extrusion2" add sketch "Sketch3" along normal blind 2.54
sketch "Sketch4" plane through (0, 0, 15.24) normal (0, 0, 1) x (1, 0, 0)
  spline S0 degree 4 poles (-34.6772, 23.4704) (-38.4839, 22.7648) (-40.4639, 22.3554) (-50.7282, 21.246) (-60.3841, 16.8007) (-62.8171, 16.4662) (-68.298, 12.2075) (-69.5248, 8.3693) (-64.0493, 2.7683) (-55.3104, -0.0117) (-47.7069, -2.169) (-33.9304, -4.8768) (-23.6731, -6.2287) (-9.6141, -6.7589) (3.746, -7.4013) (15.6562, -7.092) (30.638, -6.3684) (37.5145, -5.6068) (39.0554, -5.469) knots 0 0 0 0 0 0.119852 0.168842 0.217962 0.26068 0.302266 0.349885 0.400894 0.460541 0.525181 0.593374 0.664659 0.734215 0.804927 0.871867 1 1 1 1 1 projected
  arc A0 (39.108, -5.7709) -> (39.0554, -5.469) centre (39.0691, -5.6221) ccw projected
  spline S1 degree 4 poles (39.108, -5.7709) (37.4385, -6.308) (23.1011, -7.5786) (13.1163, -8.7313) (-7.0091, -8.2583) (-21.4952, -8.578) (-29.5439, -7.3415) (-41.2987, -6.7959) (-48.8299, -4.501) (-65.2605, -1.3176) (-67.5791, 0.1162) knots 0 0 0 0 0 0.240077 0.356564 0.466749 0.569739 0.662256 0.754281 1 1 1 1 1 projected
  spline S2 degree 4 poles (-68.0997, -0.655) (-62.5259, -3.4157) (-61.765, -4.6975) (-42.4071, -9.0657) (-34.3124, -10.69) (-17.9846, -11.881) (-11.8888, -12.3355) (4.7444, -12.3507) (10.0463, -12.6177) (17.9731, -11.9242) (19.2729, -11.797) knots 0 0 0 0 0 0.246404 0.35873 0.472789 0.584911 0.695079 0.795942 1 1 1 1 1 projected
  arc A1 (19.2729, -12.2118) -> (19.2729, -11.797) centre (19.2444, -12.0044) ccw projected
  spline S3 degree 4 poles (-52.048, 23.4288) (-54.2401, 23.3528) (-66.6857, 19.9381) (-79.4427, 16.3789) (-84.3823, 7.744) (-84.209, 4.7623) (-78.8244, -2.3227) (-66.6046, -6.5374) (-51.6417, -10.096) (-41.0552, -11.7905) (-18.7063, -14.7429) (-1.7175, -12.2275) (3.8289, -14.3334) (19.2729, -12.2118) knots 0 0 0 0 0 0.18081 0.244398 0.299004 0.356886 0.425964 0.50631 0.595714 0.686149 0.771857 1 1 1 1 1 projected
  arc A2 (-67.5791, 0.1162) -> (-68.0997, -0.655) centre (-67.7515, -0.3288) ccw projected
  arc A3 (-51.972, 22.8466) -> (-52.048, 23.4288) centre (-52.0378, 23.1341) ccw projected
  spline S4 degree 4 poles (-51.972, 22.8466) (-57.6402, 21.3754) (-58.1641, 21.4536) (-67.5415, 18.1413) (-68.4686, 17.0097) knots 0 0 0 0 0 1 1 1 1 1 projected
  spline S5 degree 4 poles (-67.7151, 16.4274) (-64.426, 17.854) (-60.1317, 19.3505) (-45.9619, 22.8498) (-40.2437, 23.0375) (-34.715, 23.8652) knots 0 0 0 0 0 0.467692 1 1 1 1 1 projected
  arc A4 (-34.6772, 23.4704) -> (-34.715, 23.8652) centre (-34.6856, 23.6688) ccw projected
  arc A5 (-68.4686, 17.0097) -> (-67.7151, 16.4274) centre (-67.9772, 16.8669) ccw
  point P0 (0, 0)
  constraints: 2 point on circle, 1 centre point
extrude "Extrusion3" add sketch "Sketch4" along normal blind 0.508
sketch "Sketch5" plane through (0, 0, 15.748) normal (0, 0, 1) x (1, 0, 0)
  spline S0 degree 4 poles (-71.97, 15.4745) (-73.5618, 14.8176) (-78.0389, 12.5988) (-80.1652, 8.5391) (-80.3177, 3.0778) (-71.7488, -2.2177) (-71.8816, -1.1731) (-68.0997, -2.6081) knots 0 0 0 0 0 0.349269 0.493319 0.634154 1 1 1 1 1 projected
  spline S1 degree 4 poles (-75.8015, 6.7353) (-75.5788, 4.044) (-75.7088, 2.5492) (-69.058, -1.4354) (-68.0997, -2.6081) knots 0 0 0 0 0 1 1 1 1 1 projected
  spline S2 degree 4 poles (-75.8015, 6.7353) (-74.6191, 4.6802) (-72.4475, 2.5037) (-68.6605, 1.822) (-66.4762, 1.8118) knots 0 0 0 0 0 1 1 1 1 1 projected
  spline S3 degree 4 poles (-69.6154, 14.6163) (-70.4759, 13.8231) (-72.3788, 12.3221) (-73.059, 10.2756) (-73.1664, 5.2191) (-69.7067, 3.7408) (-68.2199, 2.6138) (-66.4762, 1.8118) knots 0 0 0 0 0 0.339065 0.480526 0.625412 1 1 1 1 1 projected
  spline S4 degree 3 poles (-75.6158, 10.3382) (-74.6308, 12.2137) (-72.1942, 13.8735) (-69.6154, 14.6163) knots 0 0 0 0 1 1 1 1 projected
  spline S5 degree 3 poles (-71.97, 15.4745) (-73.2885, 14.039) (-75.2326, 12.8836) (-75.6158, 10.3382) knots 0 0 0 0 1 1 1 1 projected
  point P0 (0, 0)
extrude "Extrusion4" add sketch "Sketch5" along normal blind 0.508
sketch "Sketch6" plane through (0, 0, 15.24) normal (0, 0, 1) x (1, 0, 0)
  spline S0 degree 4 poles (-29.4647, 15.575) (-28.1519, 15.0835) (-24.5872, 15.8727) (-18.5009, 18.1038) (-12.5083, 20.6718) (-6.1161, 23.2421) (3.0018, 24.3814) (11.5231, 23.0257) (21.4229, 19.5107) (27.5772, 14.3886) (34.927, 6.7369) (34.8654, 5.7735) knots 0 0 0 0 0 0.174571 0.259653 0.353316 0.452487 0.556196 0.662312 0.769869 1 1 1 1 1 projected
  spline S1 degree 4 poles (34.8654, 5.7735) (40.8292, 8.1161) (40.6549, 10.0927) (71.7532, 15.7804) (83.2327, 13.7336) (92.5145, 13.0285) (96.6582, 8.6519) (94.223, 5.852) (89.2683, 3.6409) (84.9003, 2.9408) (72.4496, 1.6108) (62.4885, 0.1154) (50.6338, -0.6616) (26.6259, -2.1909) (16.6731, -2.1299) (2.2887, -2.9635) (-18.4876, -2.0158) (-30.9684, -1.9125) (-54.5772, 2.6604) (-59.4474, 3.6818) (-65.879, 9.2635) knots 0 0 0 0 0 0.126651 0.181647 0.230811 0.266967 0.298491 0.327835 0.362864 0.404742 0.452577 0.510294 0.568494 0.62822 0.690828 0.748447 0.808493 0.867431 1 1 1 1 1 projected
  spline S2 degree 4 poles (-65.879, 9.2635) (-65.8749, 11.3275) (-55.3373, 15.7109) (-53.6712, 18.2111) (-38.9955, 17.9177) (-37.405, 16.714) (-33.7493, 19.5352) (-31.3534, 18.3976) (-29.5789, 16.7809) (-29.4647, 15.575) knots 0 0 0 0 0 0.357646 0.495506 0.61467 0.716133 0.79801 1 1 1 1 1 projected
  point P0 (0, 0)
extrude "Extrusion5" add sketch "Sketch6" along normal blind 0.508
sketch "Sketch7" plane through (0, 0, 15.748) normal (0, 0, 1) x (1, 0, 0)
  spline S0 degree 3 poles (-50.0556, 11.6422) (-48.6963, 12.1055) (-46.1374, 12.8984) (-44.3311, 13.1726) knots 0 0 0 0 1 1 1 1 projected
  line L0 (-49.9017, 9.2326) -> (-50.0556, 11.6422) projected
  line L1 (-51.5889, 11.0921) -> (-49.9017, 9.2326) projected
  spline S1 degree 2 poles (-53.3008, 9.911) (-52.5867, 10.6807) (-51.5889, 11.0921) knots 0 0 0 1 1 1 projected
  spline S2 degree 4 poles (-47.2677, 11.1827) (-47.3636, 10.8042) (-47.2649, 10.0321) (-49.615, 8.1093) (-50.6841, 8.6477) (-52.7122, 9.4891) (-53.3008, 9.911) knots 0 0 0 0 0 0.361372 0.533494 1 1 1 1 1 projected
  spline S3 degree 3 poles (-44.3311, 13.1726) (-45.5318, 12.4854) (-46.2357, 11.5206) (-47.2677, 11.1827) knots 0 0 0 0 1 1 1 1 projected
  line L2 (35.2952, 4.3814) -> (36.3498, 1.9636) projected
  spline S4 degree 2 poles (35.2952, 4.3814) (37.0043, 5.036) (38.6042, 5.5033) knots 0 0 0 1 1 1 projected
  spline S5 degree 2 poles (38.6042, 5.5033) (40.0266, 5.3532) (41.2291, 4.6206) knots 0 0 0 1 1 1 projected
  spline S6 degree 2 poles (38.9714, 2.5521) (39.7159, 3.5541) (41.2291, 4.6206) knots 0 0 0 1 1 1 projected
  spline S7 degree 2 poles (36.3498, 1.9636) (37.741, 2.2189) (38.9714, 2.5521) knots 0 0 0 1 1 1 projected
  spline S8 degree 2 poles (41.6408, 3.0069) (41.951, 3.9202) (42.3855, 4.2937) knots 0 0 0 1 1 1 projected
  spline S9 degree 2 poles (42.3855, 4.2937) (43.4958, 4.1245) (44.1266, 3.4055) knots 0 0 0 1 1 1 projected
  line L3 (41.6408, 3.0069) -> (44.1266, 3.4055) projected
  spline S10 degree 2 poles (39.2749, 5.685) (40.8676, 5.5413) (42.1574, 5.2848) knots 0 0 0 1 1 1 projected
  spline S11 degree 2 poles (42.1574, 5.2848) (43.1477, 6.2989) (44.8399, 7.0186) knots 0 0 0 1 1 1 projected
  spline S12 degree 2 poles (44.8399, 7.0186) (43.7611, 6.1187) (43.1407, 5.2848) knots 0 0 0 1 1 1 projected
  spline S13 degree 3 poles (43.1407, 5.2848) (44.4101, 5.0932) (46.3814, 4.5665) (47.5565, 4.0873) knots 0 0 0 0 1 1 1 1 projected
  spline S14 degree 4 poles (39.2749, 5.685) (40.1857, 6.0134) (43.263, 7.1325) (47.2971, 8.314) (55.8577, 10.4813) (59.3016, 11.343) (70.558, 12.3008) (76.0447, 12.4509) (85.7728, 11.2662) (89.5634, 10.9909) (92.783, 8.8272) (92.8791, 7.6694) (92.0215, 6.1081) (89.9165, 5.6648) (89.4278, 5.5033) knots 0 0 0 0 0 0.162413 0.243574 0.336675 0.435958 0.540053 0.643161 0.731074 0.799741 0.849228 0.891651 1 1 1 1 1 projected
  spline S15 degree 3 poles (47.5565, 4.0873) (48.3925, 4.8563) (50.3732, 6.2541) (51.2037, 6.5341) knots 0 0 0 0 1 1 1 1 projected
  spline S16 degree 3 poles (55.7131, 8.7927) (54.9237, 8.3987) (53.6734, 7.6255) (53.2188, 7.0186) knots 0 0 0 0 1 1 1 1 projected
  spline S17 degree 3 poles (52.024, 7.099) (53.0571, 7.7103) (54.2865, 8.498) (55.7131, 8.7927) knots 0 0 0 0 1 1 1 1 projected
  spline S18 degree 3 poles (48.5739, 7.2608) (49.332, 7.5631) (51.2725, 7.4257) (52.024, 7.099) knots 0 0 0 0 1 1 1 1 projected
  spline S19 degree 3 poles (51.2037, 6.5341) (50.1722, 6.995) (49.7103, 7.113) (48.5739, 7.2608) knots 0 0 0 0 1 1 1 1 projected
  spline S20 degree 2 poles (51.5538, 4.7315) (51.7348, 5.3219) (52.4733, 6.2312) knots 0 0 0 1 1 1 projected
  spline S21 degree 2 poles (52.4733, 6.2312) (53.4059, 5.9476) (54.4025, 5.2848) knots 0 0 0 1 1 1 projected
  line L4 (51.5538, 4.7315) -> (54.4025, 5.2848) projected
  spline S22 degree 3 poles (53.2188, 7.0186) (53.9015, 6.9339) (55.7193, 6.6122) (56.9696, 5.685) knots 0 0 0 0 1 1 1 1 projected
  spline S23 degree 2 poles (56.9696, 5.685) (58.6077, 7.5518) (60.7559, 8.5077) knots 0 0 0 1 1 1 projected
  spline S24 degree 3 poles (62.5551, 8.7927) (64.4258, 8.2771) (65.688, 7.6378) (66.7581, 6.7295) knots 0 0 0 0 1 1 1 1 projected
  spline S25 degree 2 poles (60.7559, 8.5077) (59.8431, 8.9671) (58.568, 9.2635) knots 0 0 0 1 1 1 projected
  spline S26 degree 2 poles (58.568, 9.2635) (59.9688, 9.4306) (61.5188, 8.9027) knots 0 0 0 1 1 1 projected
  spline S27 degree 2 poles (61.5188, 8.9027) (62.6832, 9.7229) (64.527, 10.2202) knots 0 0 0 1 1 1 projected
  spline S28 degree 2 poles (64.527, 10.2202) (63.4518, 9.6666) (62.5551, 8.7927) knots 0 0 0 1 1 1 projected
  spline S29 degree 2 poles (61.7016, 8.0103) (63.1746, 7.5515) (63.8972, 6.3408) knots 0 0 0 1 1 1 projected
  spline S30 degree 2 poles (60.3527, 5.9944) (60.8212, 7.1738) (61.7016, 8.0103) knots 0 0 0 1 1 1 projected
  line L5 (60.3527, 5.9944) -> (63.8972, 6.3408) projected
  spline S31 degree 3 poles (66.7581, 6.7295) (67.8827, 7.847) (69.6665, 8.8024) (70.7025, 8.9027) knots 0 0 0 0 1 1 1 1 projected
  spline S32 degree 3 poles (70.7025, 8.9027) (70.1912, 9.604) (68.038, 10.1459) (66.9267, 10.338) knots 0 0 0 0 1 1 1 1 projected
  spline S33 degree 3 poles (66.9267, 10.338) (68.3767, 10.6734) (70.5215, 9.7878) (71.7293, 9.5928) knots 0 0 0 0 1 1 1 1 projected
  spline S34 degree 3 poles (71.7293, 9.5928) (72.6223, 9.9336) (74.2672, 10.8902) (75.4899, 10.9318) knots 0 0 0 0 1 1 1 1 projected
  spline S35 degree 3 poles (75.4899, 10.9318) (74.5963, 10.619) (73.0858, 9.6113) (72.8404, 9.2635) knots 0 0 0 0 1 1 1 1 projected
  spline S36 degree 3 poles (72.8404, 9.2635) (74.6153, 8.8325) (75.731, 8.1456) (77.423, 7.4588) knots 0 0 0 0 1 1 1 1 projected
  spline S37 degree 2 poles (72.0142, 8.5077) (73.1907, 8.178) (73.8247, 7.2162) knots 0 0 0 1 1 1 projected
  spline S38 degree 2 poles (70.7025, 7.1374) (71.1539, 7.9459) (72.0142, 8.5077) knots 0 0 0 1 1 1 projected
  line L6 (70.7025, 7.1374) -> (73.8247, 7.2162) projected
  spline S39 degree 3 poles (80.6667, 9.2635) (78.9368, 8.8382) (78.6712, 8.3465) (77.423, 7.4588) knots 0 0 0 0 1 1 1 1 projected
  spline S40 degree 2 poles (80.6667, 7.5944) (80.9598, 8.3322) (81.6868, 8.7444) knots 0 0 0 1 1 1 projected
  spline S41 degree 2 poles (81.6868, 8.7444) (82.2926, 8.3928) (82.8551, 7.5944) knots 0 0 0 1 1 1 projected
  line L7 (80.6667, 7.5944) -> (82.8551, 7.5944) projected
  spline S42 degree 2 poles (85.9445, 7.2852) (85.1544, 8.1452) (82.7618, 9.2635) knots 0 0 0 1 1 1 projected
  spline S43 degree 2 poles (82.7618, 9.2635) (83.5886, 10.0911) (85.0626, 10.3382) knots 0 0 0 1 1 1 projected
  spline S44 degree 2 poles (85.0626, 10.3382) (83.7496, 10.5873) (81.9313, 9.718) knots 0 0 0 1 1 1 projected
  spline S45 degree 3 poles (81.9313, 9.718) (80.9342, 10.2789) (79.3639, 10.9061) (77.8217, 11.0035) knots 0 0 0 0 1 1 1 1 projected
  spline S46 degree 3 poles (89.9993, 8.7444) (89.0353, 9.1151) (87.0785, 8.2126) (85.9445, 7.2852) knots 0 0 0 0 1 1 1 1 projected
  spline S47 degree 2 poles (87.5827, 7.1374) (88.251, 8.0136) (89.9993, 8.7444) knots 0 0 0 1 1 1 projected
  spline S48 degree 3 poles (89.4278, 5.5033) (90.0048, 6.3278) (88.6176, 6.9599) (87.5827, 7.1374) knots 0 0 0 0 1 1 1 1 projected
  spline S49 degree 3 poles (77.8217, 11.0035) (78.7555, 10.5207) (80.1921, 9.8801) (80.6667, 9.2635) knots 0 0 0 0 1 1 1 1 projected
  point P0 (0, 0)
extrude "Extrusion6" cut sketch "Sketch7" against normal blind 1.016